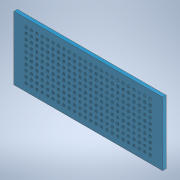
# Autodesk Inventor part: плата панели
Saved by Autodesk Inventor 2022 (Build 260153000, 153)
## iProperties
Created: 2022-06-07
Part Number: плата панели
Material: Типовые
Document SubType Name: Modeling
Designer: Admin
Density: 1 g/cm^3
Appearance: По умолчанию
Author: Admin
Autodesk Inventor part; units mm, degrees
ref_plane "YZ Plane" through (0, 0, 0) normal (1, 0, 0) x (0, 1, 0)
ref_plane "XZ Plane" through (0, 0, 0) normal (0, 1, 0) x (-1, 0, 0)
ref_plane "XY Plane" through (0, 0, 0) normal (0, 0, 1) x (1, 0, 0)
sketch "Эскиз1" plane through (0, 0, 0) normal (0, 0, 1) x (1, 0, 0)
  line L0 (-35, 15) -> (35, 15)
  line L1 (35, 15) -> (35, -15)
  line L2 (35, -15) -> (-35, -15)
  line L3 (-35, -15) -> (-35, 15)
  circle A0 centre (-29.21, 11.43) radius 0.5
  circle A1 centre (-29.21, 8.89) radius 0.5
  circle A2 centre (-29.21, 6.35) radius 0.5
  circle A3 centre (-29.21, 3.81) radius 0.5
  circle A4 centre (-29.21, 1.27) radius 0.5
  circle A5 centre (-29.21, -1.27) radius 0.5
  circle A6 centre (-29.21, -3.81) radius 0.5
  circle A7 centre (-29.21, -6.35) radius 0.5
  circle A8 centre (-29.21, -8.89) radius 0.5
  circle A9 centre (-29.21, -11.43) radius 0.5
  circle A10 centre (-26.67, 11.43) radius 0.5
  circle A11 centre (-26.67, 8.89) radius 0.5
  circle A12 centre (-26.67, 6.35) radius 0.5
  circle A13 centre (-26.67, 3.81) radius 0.5
  circle A14 centre (-26.67, 1.27) radius 0.5
  circle A15 centre (-26.67, -1.27) radius 0.5
  circle A16 centre (-26.67, -3.81) radius 0.5
  circle A17 centre (-26.67, -6.35) radius 0.5
  circle A18 centre (-26.67, -8.89) radius 0.5
  circle A19 centre (-26.67, -11.43) radius 0.5
  circle A20 centre (-24.13, 11.43) radius 0.5
  circle A21 centre (-24.13, 8.89) radius 0.5
  circle A22 centre (-24.13, 6.35) radius 0.5
  circle A23 centre (-24.13, 3.81) radius 0.5
  circle A24 centre (-24.13, 1.27) radius 0.5
  circle A25 centre (-24.13, -1.27) radius 0.5
  circle A26 centre (-24.13, -3.81) radius 0.5
  circle A27 centre (-24.13, -6.35) radius 0.5
  circle A28 centre (-24.13, -8.89) radius 0.5
  circle A29 centre (-24.13, -11.43) radius 0.5
  circle A30 centre (-21.59, 11.43) radius 0.5
  circle A31 centre (-21.59, 8.89) radius 0.5
  circle A32 centre (-21.59, 6.35) radius 0.5
  circle A33 centre (-21.59, 3.81) radius 0.5
  circle A34 centre (-21.59, 1.27) radius 0.5
  circle A35 centre (-21.59, -1.27) radius 0.5
  circle A36 centre (-21.59, -3.81) radius 0.5
  circle A37 centre (-21.59, -6.35) radius 0.5
  circle A38 centre (-21.59, -8.89) radius 0.5
  circle A39 centre (-21.59, -11.43) radius 0.5
  circle A40 centre (-19.05, 11.43) radius 0.5
  circle A41 centre (-19.05, 8.89) radius 0.5
  circle A42 centre (-19.05, 6.35) radius 0.5
  circle A43 centre (-19.05, 3.81) radius 0.5
  circle A44 centre (-19.05, 1.27) radius 0.5
  circle A45 centre (-19.05, -1.27) radius 0.5
  circle A46 centre (-19.05, -3.81) radius 0.5
  circle A47 centre (-19.05, -6.35) radius 0.5
  circle A48 centre (-19.05, -8.89) radius 0.5
  circle A49 centre (-19.05, -11.43) radius 0.5
  circle A50 centre (-16.51, 11.43) radius 0.5
  circle A51 centre (-16.51, 8.89) radius 0.5
  circle A52 centre (-16.51, 6.35) radius 0.5
  circle A53 centre (-16.51, 3.81) radius 0.5
  circle A54 centre (-16.51, 1.27) radius 0.5
  circle A55 centre (-16.51, -1.27) radius 0.5
  circle A56 centre (-16.51, -3.81) radius 0.5
  circle A57 centre (-16.51, -6.35) radius 0.5
  circle A58 centre (-16.51, -8.89) radius 0.5
  circle A59 centre (-16.51, -11.43) radius 0.5
  circle A60 centre (-13.97, 11.43) radius 0.5
  circle A61 centre (-13.97, 8.89) radius 0.5
  circle A62 centre (-13.97, 6.35) radius 0.5
  circle A63 centre (-13.97, 3.81) radius 0.5
  circle A64 centre (-13.97, 1.27) radius 0.5
  circle A65 centre (-13.97, -1.27) radius 0.5
  circle A66 centre (-13.97, -3.81) radius 0.5
  circle A67 centre (-13.97, -6.35) radius 0.5
  circle A68 centre (-13.97, -8.89) radius 0.5
  circle A69 centre (-13.97, -11.43) radius 0.5
  circle A70 centre (-11.43, 11.43) radius 0.5
  circle A71 centre (-11.43, 8.89) radius 0.5
  circle A72 centre (-11.43, 6.35) radius 0.5
  circle A73 centre (-11.43, 3.81) radius 0.5
  circle A74 centre (-11.43, 1.27) radius 0.5
  circle A75 centre (-11.43, -1.27) radius 0.5
  circle A76 centre (-11.43, -3.81) radius 0.5
  circle A77 centre (-11.43, -6.35) radius 0.5
  circle A78 centre (-11.43, -8.89) radius 0.5
  circle A79 centre (-11.43, -11.43) radius 0.5
  circle A80 centre (-8.89, 11.43) radius 0.5
  circle A81 centre (-8.89, 8.89) radius 0.5
  circle A82 centre (-8.89, 6.35) radius 0.5
  circle A83 centre (-8.89, 3.81) radius 0.5
  circle A84 centre (-8.89, 1.27) radius 0.5
  circle A85 centre (-8.89, -1.27) radius 0.5
  circle A86 centre (-8.89, -3.81) radius 0.5
  circle A87 centre (-8.89, -6.35) radius 0.5
  circle A88 centre (-8.89, -8.89) radius 0.5
  circle A89 centre (-8.89, -11.43) radius 0.5
  circle A90 centre (-6.35, 11.43) radius 0.5
  circle A91 centre (-6.35, 8.89) radius 0.5
  circle A92 centre (-6.35, 6.35) radius 0.5
  circle A93 centre (-6.35, 3.81) radius 0.5
  circle A94 centre (-6.35, 1.27) radius 0.5
  circle A95 centre (-6.35, -1.27) radius 0.5
  circle A96 centre (-6.35, -3.81) radius 0.5
  circle A97 centre (-6.35, -6.35) radius 0.5
  circle A98 centre (-6.35, -8.89) radius 0.5
  circle A99 centre (-6.35, -11.43) radius 0.5
  circle A100 centre (-3.81, 11.43) radius 0.5
  circle A101 centre (-3.81, 8.89) radius 0.5
  circle A102 centre (-3.81, 6.35) radius 0.5
  circle A103 centre (-3.81, 3.81) radius 0.5
  circle A104 centre (-3.81, 1.27) radius 0.5
  circle A105 centre (-3.81, -1.27) radius 0.5
  circle A106 centre (-3.81, -3.81) radius 0.5
  circle A107 centre (-3.81, -6.35) radius 0.5
  circle A108 centre (-3.81, -8.89) radius 0.5
  circle A109 centre (-3.81, -11.43) radius 0.5
  circle A110 centre (-1.27, 11.43) radius 0.5
  circle A111 centre (-1.27, 8.89) radius 0.5
  circle A112 centre (-1.27, 6.35) radius 0.5
  circle A113 centre (-1.27, 3.81) radius 0.5
  circle A114 centre (-1.27, 1.27) radius 0.5
  circle A115 centre (-1.27, -1.27) radius 0.5
  circle A116 centre (-1.27, -3.81) radius 0.5
  circle A117 centre (-1.27, -6.35) radius 0.5
  circle A118 centre (-1.27, -8.89) radius 0.5
  circle A119 centre (-1.27, -11.43) radius 0.5
  circle A120 centre (1.27, 11.43) radius 0.5
  circle A121 centre (1.27, 8.89) radius 0.5
  circle A122 centre (1.27, 6.35) radius 0.5
  circle A123 centre (1.27, 3.81) radius 0.5
  circle A124 centre (1.27, 1.27) radius 0.5
  circle A125 centre (1.27, -1.27) radius 0.5
  circle A126 centre (1.27, -3.81) radius 0.5
  circle A127 centre (1.27, -6.35) radius 0.5
  circle A128 centre (1.27, -8.89) radius 0.5
  circle A129 centre (1.27, -11.43) radius 0.5
  circle A130 centre (3.81, 11.43) radius 0.5
  circle A131 centre (3.81, 8.89) radius 0.5
  circle A132 centre (3.81, 6.35) radius 0.5
  circle A133 centre (3.81, 3.81) radius 0.5
  circle A134 centre (3.81, 1.27) radius 0.5
  circle A135 centre (3.81, -1.27) radius 0.5
  circle A136 centre (3.81, -3.81) radius 0.5
  circle A137 centre (3.81, -6.35) radius 0.5
  circle A138 centre (3.81, -8.89) radius 0.5
  circle A139 centre (3.81, -11.43) radius 0.5
  circle A140 centre (6.35, 11.43) radius 0.5
  circle A141 centre (6.35, 8.89) radius 0.5
  circle A142 centre (6.35, 6.35) radius 0.5
  circle A143 centre (6.35, 3.81) radius 0.5
  circle A144 centre (6.35, 1.27) radius 0.5
  circle A145 centre (6.35, -1.27) radius 0.5
  circle A146 centre (6.35, -3.81) radius 0.5
  circle A147 centre (6.35, -6.35) radius 0.5
  circle A148 centre (6.35, -8.89) radius 0.5
  circle A149 centre (6.35, -11.43) radius 0.5
  circle A150 centre (8.89, 11.43) radius 0.5
  circle A151 centre (8.89, 8.89) radius 0.5
  circle A152 centre (8.89, 6.35) radius 0.5
  circle A153 centre (8.89, 3.81) radius 0.5
  circle A154 centre (8.89, 1.27) radius 0.5
  circle A155 centre (8.89, -1.27) radius 0.5
  circle A156 centre (8.89, -3.81) radius 0.5
  circle A157 centre (8.89, -6.35) radius 0.5
  circle A158 centre (8.89, -8.89) radius 0.5
  circle A159 centre (8.89, -11.43) radius 0.5
  circle A160 centre (11.43, 11.43) radius 0.5
  circle A161 centre (11.43, 8.89) radius 0.5
  circle A162 centre (11.43, 6.35) radius 0.5
  circle A163 centre (11.43, 3.81) radius 0.5
  circle A164 centre (11.43, 1.27) radius 0.5
  circle A165 centre (11.43, -1.27) radius 0.5
  circle A166 centre (11.43, -3.81) radius 0.5
  circle A167 centre (11.43, -6.35) radius 0.5
  circle A168 centre (11.43, -8.89) radius 0.5
  circle A169 centre (11.43, -11.43) radius 0.5
  circle A170 centre (13.97, 11.43) radius 0.5
  circle A171 centre (13.97, 8.89) radius 0.5
  circle A172 centre (13.97, 6.35) radius 0.5
  circle A173 centre (13.97, 3.81) radius 0.5
  circle A174 centre (13.97, 1.27) radius 0.5
  circle A175 centre (13.97, -1.27) radius 0.5
  circle A176 centre (13.97, -3.81) radius 0.5
  circle A177 centre (13.97, -6.35) radius 0.5
  circle A178 centre (13.97, -8.89) radius 0.5
  circle A179 centre (13.97, -11.43) radius 0.5
  circle A180 centre (16.51, 11.43) radius 0.5
  circle A181 centre (16.51, 8.89) radius 0.5
  circle A182 centre (16.51, 6.35) radius 0.5
  circle A183 centre (16.51, 3.81) radius 0.5
  circle A184 centre (16.51, 1.27) radius 0.5
  circle A185 centre (16.51, -1.27) radius 0.5
  circle A186 centre (16.51, -3.81) radius 0.5
  circle A187 centre (16.51, -6.35) radius 0.5
  circle A188 centre (16.51, -8.89) radius 0.5
  circle A189 centre (16.51, -11.43) radius 0.5
  circle A190 centre (19.05, 11.43) radius 0.5
  circle A191 centre (19.05, 8.89) radius 0.5
  circle A192 centre (19.05, 6.35) radius 0.5
  circle A193 centre (19.05, 3.81) radius 0.5
  circle A194 centre (19.05, 1.27) radius 0.5
  circle A195 centre (19.05, -1.27) radius 0.5
  circle A196 centre (19.05, -3.81) radius 0.5
  circle A197 centre (19.05, -6.35) radius 0.5
  circle A198 centre (19.05, -8.89) radius 0.5
  circle A199 centre (19.05, -11.43) radius 0.5
  circle A200 centre (21.59, 11.43) radius 0.5
  circle A201 centre (21.59, 8.89) radius 0.5
  circle A202 centre (21.59, 6.35) radius 0.5
  circle A203 centre (21.59, 3.81) radius 0.5
  circle A204 centre (21.59, 1.27) radius 0.5
  circle A205 centre (21.59, -1.27) radius 0.5
  circle A206 centre (21.59, -3.81) radius 0.5
  circle A207 centre (21.59, -6.35) radius 0.5
  circle A208 centre (21.59, -8.89) radius 0.5
  circle A209 centre (21.59, -11.43) radius 0.5
  circle A210 centre (24.13, 11.43) radius 0.5
  circle A211 centre (24.13, 8.89) radius 0.5
  circle A212 centre (24.13, 6.35) radius 0.5
  circle A213 centre (24.13, 3.81) radius 0.5
  circle A214 centre (24.13, 1.27) radius 0.5
  circle A215 centre (24.13, -1.27) radius 0.5
  circle A216 centre (24.13, -3.81) radius 0.5
  circle A217 centre (24.13, -6.35) radius 0.5
  circle A218 centre (24.13, -8.89) radius 0.5
  circle A219 centre (24.13, -11.43) radius 0.5
  circle A220 centre (26.67, 11.43) radius 0.5
  circle A221 centre (26.67, 8.89) radius 0.5
  circle A222 centre (26.67, 6.35) radius 0.5
  circle A223 centre (26.67, 3.81) radius 0.5
  circle A224 centre (26.67, 1.27) radius 0.5
  circle A225 centre (26.67, -1.27) radius 0.5
  circle A226 centre (26.67, -3.81) radius 0.5
  circle A227 centre (26.67, -6.35) radius 0.5
  circle A228 centre (26.67, -8.89) radius 0.5
  circle A229 centre (26.67, -11.43) radius 0.5
  circle A230 centre (29.21, 11.43) radius 0.5
  circle A231 centre (29.21, 8.89) radius 0.5
  circle A232 centre (29.21, 6.35) radius 0.5
  circle A233 centre (29.21, 3.81) radius 0.5
  circle A234 centre (29.21, 1.27) radius 0.5
  circle A235 centre (29.21, -1.27) radius 0.5
  circle A236 centre (29.21, -3.81) radius 0.5
  circle A237 centre (29.21, -6.35) radius 0.5
  circle A238 centre (29.21, -8.89) radius 0.5
  circle A239 centre (29.21, -11.43) radius 0.5
  line L4 (0, 15) -> (0, -15)
  line L5 (35, 0) -> (-35, 0)
  point P0 (0, 0)
  point P1 (-26.67, 0)
  point P2 (-6.35, 0)
  dimension "d0" = 30
  dimension "d1" = 70
  dimension "d2" = 1
  dimension "d5" = 2.54
  dimension "d8" = 2.54
  constraints: 240 centre point, 12 end point, 4 midpoint, 3 vertical alignment, 2 horizontal, 2 parallel, 2 point on line, 1 horizontal alignment, 1 perpendicular, 1 vertical, 480 other
  measures "d0" distance of L0.end L1.end
  measures "d1" distance of L0.start L0.end
  measures "d2" diameter of A0
  measures "d5" distance of A0.centre A1.centre
  measures "d8" distance of A0.centre A10.centre
extrude "Выдавливание1" add sketch "Эскиз1" along normal blind 1.6
sketch "Эскиз2" plane through (0, 0, 0) normal (0, 0, -1) x (1, 0, 0)
  point P0 (0, 0)
  point P1 (-26.67, 0)
  point P2 (-6.35, 0)
  point P3 (-16.51, -8.89)
  point P4 (-16.51, 8.89)
